Autodesk Fusion 360 part; units mm, degrees
(part 3 of 3)
sketch "Sketch29" plane through (0, 0, 0) normal (0, -1, 0) x (1, 0, 0)
  circle A0 centre (45.8848, 89.005) radius 3.5
  circle A1 centre (45.9348, 29.975) radius 3.5
  line L0 (54.755, 44.6) -> (66.755, 44.6)
  line L1 (66.755, 44.6) -> (66.755, 32.6)
  line L2 (66.755, 32.6) -> (54.755, 32.6)
  line L3 (54.755, 32.6) -> (54.755, 44.6)
  line L4 (2.5, 100.965) -> (2.5, 17.885)
  line L5 (2.5, 17.885) -> (83.65, 17.885)
  line L6 (83.65, 17.885) -> (83.65, 100.965)
  line L7 (83.65, 100.965) -> (2.5, 100.965)
  line L8 (48.98, 56.225) -> (48.98, 85.865)
  line L9 (48.98, 85.865) -> (66.9, 85.865)
  line L10 (66.9, 85.865) -> (66.9, 56.225)
  line L11 (66.9, 56.225) -> (48.98, 56.225)
  circle A2 centre (74.9435, 29.945) radius 3.5
  circle A3 centre (75.1296, 88.925) radius 3.5
  line L12 (21.48, 37.8592) -> (7.48, 37.8592)
  line L13 (7.48, 37.8592) -> (7.48, 23.8592)
  line L14 (7.48, 23.8592) -> (21.48, 23.8592)
  line L15 (21.48, 23.8592) -> (21.48, 37.8592)
  line L16 (21.48, 37.8592) -> (7.48, 23.8592) construction
  line L17 (7.48, 37.8592) -> (21.48, 23.8592) construction
  line L18 (2.5, 17.885) -> (7.5, 17.885)
  line L19 (14.48, 30.8592) -> (14.48, 49.9092)
  line L20 (14.48, 49.9092) -> (14.48, 68.9592)
  line L21 (14.48, 68.9592) -> (14.48, 88.0092)
  line L22 (14.48, 88.0092) -> (33.53, 88.0092)
  line L23 (33.53, 88.0092) -> (33.53, 68.9592)
  line L24 (33.53, 68.9592) -> (33.53, 49.9092)
  line L25 (33.53, 49.9092) -> (33.53, 30.8592)
  line L26 (21.48, 56.9092) -> (7.48, 56.9092)
  line L27 (7.48, 56.9092) -> (7.48, 42.9092)
  line L28 (7.48, 42.9092) -> (21.48, 42.9092)
  line L29 (21.48, 42.9092) -> (21.48, 56.9092)
  line L30 (21.48, 56.9092) -> (7.48, 42.9092) construction
  line L31 (7.48, 56.9092) -> (21.48, 42.9092) construction
  line L32 (21.48, 75.9592) -> (7.48, 75.9592)
  line L33 (7.48, 75.9592) -> (7.48, 61.9592)
  line L34 (7.48, 61.9592) -> (21.48, 61.9592)
  line L35 (21.48, 61.9592) -> (21.48, 75.9592)
  line L36 (21.48, 75.9592) -> (7.48, 61.9592) construction
  line L37 (7.48, 75.9592) -> (21.48, 61.9592) construction
  line L38 (21.48, 95.0092) -> (7.48, 95.0092)
  line L39 (7.48, 95.0092) -> (7.48, 81.0092)
  line L40 (7.48, 81.0092) -> (21.48, 81.0092)
  line L41 (21.48, 81.0092) -> (21.48, 95.0092)
  line L42 (21.48, 95.0092) -> (7.48, 81.0092) construction
  line L43 (7.48, 95.0092) -> (21.48, 81.0092) construction
  line L44 (13.866, 17.885) -> (13.866, 23.885)
  line L45 (11.5637, 100.965) -> (11.5637, 94.965)
  line L46 (40.53, 95.0092) -> (26.53, 95.0092)
  line L47 (26.53, 95.0092) -> (26.53, 81.0092)
  line L48 (26.53, 81.0092) -> (40.53, 81.0092)
  line L49 (40.53, 81.0092) -> (40.53, 95.0092)
  line L50 (40.53, 95.0092) -> (26.53, 81.0092) construction
  line L51 (26.53, 95.0092) -> (40.53, 81.0092) construction
  line L52 (40.53, 75.9592) -> (26.53, 75.9592)
  line L53 (26.53, 75.9592) -> (26.53, 61.9592)
  line L54 (26.53, 61.9592) -> (40.53, 61.9592)
  line L55 (40.53, 61.9592) -> (40.53, 75.9592)
  line L56 (40.53, 75.9592) -> (26.53, 61.9592) construction
  line L57 (26.53, 75.9592) -> (40.53, 61.9592) construction
  line L58 (40.53, 56.9092) -> (26.53, 56.9092)
  line L59 (26.53, 56.9092) -> (26.53, 42.9092)
  line L60 (26.53, 42.9092) -> (40.53, 42.9092)
  line L61 (40.53, 42.9092) -> (40.53, 56.9092)
  line L62 (40.53, 56.9092) -> (26.53, 42.9092) construction
  line L63 (26.53, 56.9092) -> (40.53, 42.9092) construction
  line L64 (40.53, 37.8592) -> (26.53, 37.8592)
  line L65 (26.53, 37.8592) -> (26.53, 23.8592)
  line L66 (26.53, 23.8592) -> (40.53, 23.8592)
  line L67 (40.53, 23.8592) -> (40.53, 37.8592)
  line L68 (40.53, 37.8592) -> (26.53, 23.8592) construction
  line L69 (26.53, 37.8592) -> (40.53, 23.8592) construction
  point P0 (14.48, 30.8592)
  point P1 (14.48, 49.9092)
  point P2 (14.48, 68.9592)
  point P3 (14.48, 88.0092)
  point P4 (33.53, 88.0092)
  point P5 (33.53, 68.9592)
  point P6 (33.53, 49.9092)
  point P7 (33.53, 30.8592)
  dimension "d272" = 14
  dimension "d273" = 5
  dimension "d275" = 19.05
  dimension "d276" = 19.05
  dimension "d277" = 19.05
  dimension "d278" = 19.05
  dimension "d279" = 19.05
  dimension "d280" = 19.05
  dimension "d281" = 19.05
  dimension "d282" = 14
  dimension "d283" = 14
  dimension "d284" = 14
  dimension "d285" = 14
  dimension "d286" = 14
  dimension "d287" = 14
  dimension "d288" = 6
  dimension "d289" = 6
  dimension "d290" = 14
  dimension "d291" = 14
  dimension "d292" = 14
  dimension "d293" = 14
  dimension "d294" = 14
  dimension "d295" = 14
  dimension "d296" = 14
  dimension "d297" = 14
  constraint horizontal L12
  constraint perpendicular L12 L13
  constraint parallel L12 L14
  constraint parallel L13 L15
  constraint coincident L16 P0
  constraint coincident L17 P0
  constraint coincident L4.end L5.start
  constraint perpendicular L4 L18
  constraint coincident P0 L19.start
  constraint vertical L19
  constraint perpendicular L12 L20
  constraint perpendicular L12 L21
  constraint perpendicular L21 L22
  constraint perpendicular L22 L23
  constraint perpendicular L22 L24
  constraint perpendicular L22 L25
  constraint horizontal L26
  constraint perpendicular L26 L27
  constraint parallel L26 L28
  constraint parallel L27 L29
  constraint coincident L30 P1
  constraint coincident L31 P1
  constraint coincident P1 L19.end
  constraint horizontal L32
  constraint perpendicular L32 L33
  constraint parallel L32 L34
  constraint parallel L33 L35
  constraint coincident L36 P2
  constraint coincident L37 P2
  constraint coincident P2 L20.end
  constraint horizontal L38
  constraint perpendicular L38 L39
  constraint parallel L38 L40
  constraint parallel L39 L41
  constraint coincident L42 P3
  constraint coincident L43 P3
  constraint coincident P3 L21.end
  constraint coincident L5 L44.start
  constraint perpendicular L5 L44
  constraint coincident L7 L45.start
  constraint perpendicular L7 L45
  constraint horizontal L46
  constraint perpendicular L46 L47
  constraint parallel L46 L48
  constraint parallel L47 L49
  constraint coincident L50 P4
  constraint coincident L51 P4
  constraint coincident P4 L22.end
  constraint horizontal L52
  constraint perpendicular L52 L53
  constraint parallel L52 L54
  constraint parallel L53 L55
  constraint coincident L56 P5
  constraint coincident L57 P5
  constraint coincident P5 L23.end
  constraint horizontal L58
  constraint perpendicular L58 L59
  constraint parallel L58 L60
  constraint parallel L59 L61
  constraint coincident L62 P6
  constraint coincident L63 P6
  constraint coincident P6 L24.end
  constraint horizontal L64
  constraint perpendicular L64 L65
  constraint parallel L64 L66
  constraint parallel L65 L67
  constraint coincident L68 P7
  constraint coincident L69 P7
  constraint coincident P7 L25.end
  measures "d272" distance of L12.end L13.end
  measures "d273" distance of L4.end L18.end
  measures "d275" distance of P0 P1
  measures "d276" distance of P1 P2
  measures "d277" distance of P2 P3
  measures "d278" distance of P3 P4
  measures "d279" distance of P4 P5
  measures "d280" distance of P5 P6
  measures "d281" distance of P6 P7
  measures "d282" distance of L27.end L28.end
  measures "d283" distance of L26.end L27.end
  measures "d284" distance of L33.end L34.end
  measures "d285" distance of L32.end L33.end
  measures "d286" distance of L39.end L40.end
  measures "d287" distance of L38.end L39.end
  measures "d288" distance of L44.start L44.end
  measures "d289" distance of L45.start L45.end
  measures "d290" distance of L47.end L48.end
  measures "d291" distance of L46.end L47.end
  measures "d292" distance of L53.end L54.end
  measures "d293" distance of L52.end L53.end
  measures "d294" distance of L59.end L60.end
  measures "d295" distance of L58.end L59.end
  measures "d296" distance of L65.end L66.end
  measures "d297" distance of L64.end L65.end
extrude "Extrude48" cut sketch "Sketch29" against normal blind 4 contours L21 L22 L38 L39 L40 L41 | L12 L13 L14 L15 | L21 L22 L40 L41 | L20 L21 L32 L34 L35 | L20 L21 L32 L33 L34 | L19 L20 L26 L27 L28 | L19 L20 L26 L28 L29 | L22 L23 L46 L47 L48 L49 | L22 L23 L47 L48 | L23 L24 L52 L54 L55 | L23 L24 L52 L53 L54 | L24 L25 L58 L60 L61 | L24 L25 L58 L59 L60 | L64 L65 L66 L67
sketch "Sketch30" plane through (0, 0, 0) normal (0, -1, 0) x (1, 0, 0)
  circle A0 centre (75.1296, 88.925) radius 3.5
  circle A1 centre (74.9435, 29.945) radius 3.5
  line L0 (48.98, 56.225) -> (48.98, 85.865)
  line L1 (48.98, 85.865) -> (66.9, 85.865)
  line L2 (66.9, 85.865) -> (66.9, 56.225)
  line L3 (66.9, 56.225) -> (48.98, 56.225)
  line L4 (2.5, 100.965) -> (2.5, 17.885)
  line L5 (2.5, 17.885) -> (83.65, 17.885)
  line L6 (83.65, 17.885) -> (83.65, 100.965)
  line L7 (83.65, 100.965) -> (2.5, 100.965)
  line L8 (54.755, 44.6) -> (66.755, 44.6)
  line L9 (66.755, 44.6) -> (66.755, 32.6)
  line L10 (66.755, 32.6) -> (54.755, 32.6)
  line L11 (54.755, 32.6) -> (54.755, 44.6)
  circle A2 centre (45.9348, 29.975) radius 3.5
  circle A3 centre (45.8848, 89.005) radius 3.5
  line L12 (7.48, 37.8592) -> (21.48, 37.8592)
  line L13 (21.48, 37.8592) -> (21.48, 23.8592)
  line L14 (21.48, 23.8592) -> (7.48, 23.8592)
  line L15 (7.48, 23.8592) -> (7.48, 37.8592)
  line L16 (26.53, 95.0092) -> (40.53, 95.0092)
  line L17 (40.53, 95.0092) -> (40.53, 81.0092)
  line L18 (40.53, 81.0092) -> (26.53, 81.0092)
  line L19 (26.53, 81.0092) -> (26.53, 95.0092)
  line L20 (26.53, 37.8592) -> (40.53, 37.8592)
  line L21 (40.53, 37.8592) -> (40.53, 23.8592)
  line L22 (40.53, 23.8592) -> (26.53, 23.8592)
  line L23 (26.53, 23.8592) -> (26.53, 37.8592)
  line L24 (7.48, 95.0092) -> (21.48, 95.0092)
  line L25 (21.48, 95.0092) -> (21.48, 81.0092)
  line L26 (21.48, 81.0092) -> (7.48, 81.0092)
  line L27 (7.48, 81.0092) -> (7.48, 95.0092)
  line L28 (7.48, 56.9092) -> (21.48, 56.9092)
  line L29 (21.48, 56.9092) -> (21.48, 42.9092)
  line L30 (21.48, 42.9092) -> (7.48, 42.9092)
  line L31 (7.48, 42.9092) -> (7.48, 56.9092)
  line L32 (26.53, 75.9592) -> (40.53, 75.9592)
  line L33 (40.53, 75.9592) -> (40.53, 61.9592)
  line L34 (40.53, 61.9592) -> (26.53, 61.9592)
  line L35 (26.53, 61.9592) -> (26.53, 75.9592)
  line L36 (26.53, 56.9092) -> (40.53, 56.9092)
  line L37 (40.53, 56.9092) -> (40.53, 42.9092)
  line L38 (40.53, 42.9092) -> (26.53, 42.9092)
  line L39 (26.53, 42.9092) -> (26.53, 56.9092)
  line L40 (7.48, 75.9592) -> (21.48, 75.9592)
  line L41 (21.48, 75.9592) -> (21.48, 61.9592)
  line L42 (21.48, 61.9592) -> (7.48, 61.9592)
  line L43 (7.48, 61.9592) -> (7.48, 75.9592)
  line L44 (83.65, 17.885) -> (83.65, 21.885)
  line L45 (83.65, 21.885) -> (79.65, 21.885)
  circle A4 centre (79.65, 21.885) radius 4
  line L46 (83.65, 100.965) -> (79.65, 100.965)
  line L47 (79.65, 100.965) -> (79.65, 96.965)
  circle A5 centre (79.65, 96.965) radius 4
  line L48 (2.5, 100.965) -> (2.5, 96.965)
  line L49 (2.5, 96.965) -> (6.5, 96.965)
  circle A6 centre (6.5, 96.965) radius 4
  line L50 (2.5, 17.885) -> (2.5, 21.885)
  line L51 (2.5, 21.885) -> (6.5, 21.885)
  circle A7 centre (6.5, 21.885) radius 4
  line L52 (2.5, 17.885) -> (5.5, 17.885)
  line L53 (5.5, 17.885) -> (5.5, 20.885)
  circle A8 centre (5.5, 20.885) radius 1
  line L54 (83.65, 17.885) -> (80.65, 17.885)
  line L55 (80.65, 17.885) -> (80.65, 20.885)
  circle A9 centre (80.65, 20.885) radius 1
  line L56 (83.65, 100.965) -> (83.65, 97.965)
  line L57 (83.65, 97.965) -> (80.65, 97.965)
  circle A10 centre (80.65, 97.965) radius 1
  line L58 (2.5, 100.965) -> (2.5, 97.965)
  line L59 (2.5, 97.965) -> (5.5, 97.965)
  circle A11 centre (5.5, 97.965) radius 1
  dimension "d300" = 4
  dimension "d301" = 4
  dimension "d302" = 8
  dimension "d303" = 4
  dimension "d304" = 4
  dimension "d305" = 8
  dimension "d306" = 4
  dimension "d307" = 4
  dimension "d308" = 8
  dimension "d309" = 4
  dimension "d310" = 4
  dimension "d311" = 8
  dimension "d312" = 3
  dimension "d313" = 3
  dimension "d314" = 2
  dimension "d315" = 3
  dimension "d316" = 3
  dimension "d317" = 2
  dimension "d318" = 3
  dimension "d319" = 3
  dimension "d320" = 2
  dimension "d321" = 3
  dimension "d322" = 3
  dimension "d323" = 2
  constraint coincident L5.end L6.start
  constraint perpendicular L5 L44
  constraint perpendicular L6 L45
  constraint coincident L45.end A4.centre
  constraint coincident L6.end L7.start
  constraint perpendicular L6 L46
  constraint perpendicular L7 L47
  constraint coincident L47.end A5.centre
  constraint coincident L4.start L7.end
  constraint perpendicular L7 L48
  constraint perpendicular L4 L49
  constraint coincident L49.end A6.centre
  constraint coincident L4.end L5.start
  constraint perpendicular L5 L50
  constraint perpendicular L50 L51
  constraint coincident L51.end A7.centre
  constraint perpendicular L50 L52
  constraint perpendicular L52 L53
  constraint coincident L53.end A8.centre
  constraint perpendicular L44 L54
  constraint perpendicular L5 L55
  constraint coincident L55.end A9.centre
  constraint perpendicular L46 L56
  constraint perpendicular L56 L57
  constraint coincident L57.end A10.centre
  constraint perpendicular L7 L58
  constraint perpendicular L48 L59
  constraint coincident L59.end A11.centre
  measures "d300" distance of L5.end L44.end
  measures "d301" distance of L44.end L45.end
  measures "d302" diameter of A4
  measures "d303" distance of L6.end L46.end
  measures "d304" distance of L46.end L47.end
  measures "d305" diameter of A5
  measures "d306" distance of L4.start L48.end
  measures "d307" distance of L48.end L49.end
  measures "d308" diameter of A6
  measures "d309" distance of L4.end L50.end
  measures "d310" distance of L50.end L51.end
  measures "d311" diameter of A7
  measures "d312" distance of L4.end L52.end
  measures "d313" distance of L52.end L53.end
  measures "d314" diameter of A8
  measures "d315" distance of L5.end L54.end
  measures "d316" distance of L54.end L55.end
  measures "d317" diameter of A9
  measures "d318" distance of L6.end L56.end
  measures "d319" distance of L56.end L57.end
  measures "d320" diameter of A10
  measures "d321" distance of L4.start L58.end
  measures "d322" distance of L58.end L59.end
  measures "d323" diameter of A11
extrude "Extrude49" cut sketch "Sketch30" against normal blind 8 contours L4 L7 L48 A6 L58 L59 | L4 L48 A6 L59 | L6 L7 L46 A5 L56 L57 | L4 L5 L50 A7 L52 L53 | A11 | A10 | L6 A5 L57 | A8 | L5 A7 L53 | L5 L6 L44 A4 L54 L55 | A9 | L5 A4 L55
sketch "Sketch31" plane through (0, 0, 0) normal (0, -1, 0) x (1, 0, 0)
  arc A0 (79.65, 17.885) -> (83.65, 21.885) centre (79.65, 21.885) ccw
  line L0 (83.65, 21.885) -> (83.65, 96.965)
  arc A1 (83.65, 96.965) -> (79.65, 100.965) centre (79.65, 96.965) ccw
  line L1 (79.65, 100.965) -> (6.5, 100.965)
  arc A2 (6.5, 100.965) -> (2.5, 96.965) centre (6.5, 96.965) ccw
  line L2 (2.5, 96.965) -> (2.5, 21.885)
  arc A3 (2.5, 21.885) -> (6.5, 17.885) centre (6.5, 21.885) ccw
  line L3 (6.5, 17.885) -> (79.65, 17.885)
  line L4 (7.48, 75.9592) -> (21.48, 75.9592)
  line L5 (21.48, 75.9592) -> (21.48, 61.9592)
  line L6 (21.48, 61.9592) -> (7.48, 61.9592)
  line L7 (7.48, 61.9592) -> (7.48, 75.9592)
  line L8 (26.53, 56.9092) -> (40.53, 56.9092)
  line L9 (40.53, 56.9092) -> (40.53, 42.9092)
  line L10 (40.53, 42.9092) -> (26.53, 42.9092)
  line L11 (26.53, 42.9092) -> (26.53, 56.9092)
  line L12 (26.53, 75.9592) -> (40.53, 75.9592)
  line L13 (40.53, 75.9592) -> (40.53, 61.9592)
  line L14 (40.53, 61.9592) -> (26.53, 61.9592)
  line L15 (26.53, 61.9592) -> (26.53, 75.9592)
  line L16 (7.48, 56.9092) -> (21.48, 56.9092)
  line L17 (21.48, 56.9092) -> (21.48, 42.9092)
  line L18 (21.48, 42.9092) -> (7.48, 42.9092)
  line L19 (7.48, 42.9092) -> (7.48, 56.9092)
  line L20 (7.48, 95.0092) -> (21.48, 95.0092)
  line L21 (21.48, 95.0092) -> (21.48, 81.0092)
  line L22 (21.48, 81.0092) -> (7.48, 81.0092)
  line L23 (7.48, 81.0092) -> (7.48, 95.0092)
  line L24 (26.53, 37.8592) -> (40.53, 37.8592)
  line L25 (40.53, 37.8592) -> (40.53, 23.8592)
  line L26 (40.53, 23.8592) -> (26.53, 23.8592)
  line L27 (26.53, 23.8592) -> (26.53, 37.8592)
  line L28 (26.53, 95.0092) -> (40.53, 95.0092)
  line L29 (40.53, 95.0092) -> (40.53, 81.0092)
  line L30 (40.53, 81.0092) -> (26.53, 81.0092)
  line L31 (26.53, 81.0092) -> (26.53, 95.0092)
  line L32 (7.48, 37.8592) -> (21.48, 37.8592)
  line L33 (21.48, 37.8592) -> (21.48, 23.8592)
  line L34 (21.48, 23.8592) -> (7.48, 23.8592)
  line L35 (7.48, 23.8592) -> (7.48, 37.8592)
  circle A4 centre (45.8848, 89.005) radius 3.5
  circle A5 centre (45.9348, 29.975) radius 3.5
  line L36 (54.755, 44.6) -> (66.755, 44.6)
  line L37 (66.755, 44.6) -> (66.755, 32.6)
  line L38 (66.755, 32.6) -> (54.755, 32.6)
  line L39 (54.755, 32.6) -> (54.755, 44.6)
  line L40 (48.98, 56.225) -> (48.98, 85.865)
  line L41 (48.98, 85.865) -> (66.9, 85.865)
  line L42 (66.9, 85.865) -> (66.9, 56.225)
  line L43 (66.9, 56.225) -> (48.98, 56.225)
  circle A6 centre (74.9435, 29.945) radius 3.5
  circle A7 centre (75.1296, 88.925) radius 3.5
  circle A8 centre (5.5, 20.885) radius 1
  circle A9 centre (80.65, 20.885) radius 1
  circle A10 centre (80.65, 97.965) radius 1
  circle A11 centre (5.5, 97.965) radius 1
  line L44 (48.98, 56.225) -> (48.98, 54.725)
  line L45 (48.98, 54.725) -> (47.48, 54.725)
  line L46 (66.9, 85.865) -> (66.9, 87.365)
  line L47 (66.9, 87.365) -> (68.4, 87.365)
  line L48 (68.4, 87.365) -> (47.48, 87.365)
  line L49 (47.48, 87.365) -> (47.48, 54.725)
  line L50 (47.48, 54.725) -> (68.4, 54.725)
  line L51 (68.4, 54.725) -> (68.4, 87.365)
  dimension "d326" = 1.5
  dimension "d327" = 1.5
  dimension "d328" = 1.5
  dimension "d329" = 1.5
  constraint coincident L40.start L43.end
  constraint perpendicular L43 L44
  constraint perpendicular L44 L45
  constraint coincident L41.end L42.start
  constraint perpendicular L41 L46
  constraint perpendicular L46 L47
  constraint horizontal L48
  constraint vertical L49
  constraint horizontal L50
  constraint vertical L51
  measures "d326" distance of L40.start L44.end
  measures "d327" distance of L44.end L45.end
  measures "d328" distance of L41.end L46.end
  measures "d329" distance of L46.end L47.end
extrude "Extrude50" add sketch "Sketch31" along normal blind 1 contours A4 L40 L41 L44 L45 L46 L48 L49 L50 | L42 L43 L44 L46 L47 L48 L50 L51
